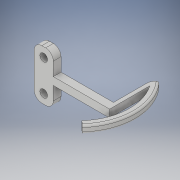
# Autodesk Inventor part: 14HM08 Chassis Sleds
Saved by Autodesk Inventor 2019 (Build 230136000, 136)
## iProperties
Created: 2019-02-17
Part Number: 14HM08 Chassis Sleds
Material: Generic
Document SubType Name: Modeling
Designer: Billy
Density: 1 g/cm^3
Appearance: Default
Author: Billy
Autodesk Inventor part; units mm, degrees
ref_plane "YZ Plane" through (0, 0, 0) normal (1, 0, 0) x (0, 1, 0)
ref_plane "XZ Plane" through (0, 0, 0) normal (0, 1, 0) x (-1, 0, 0)
ref_plane "XY Plane" through (0, 0, 0) normal (0, 0, 1) x (1, 0, 0)
sketch "Sketch1" plane through (0, 0, 0) normal (0, 1, 0) x (-1, 0, 0)
  arc A0 (-22.3607, 20) -> (-22.3607, -20) centre (0, 0) ccw
  arc A1 (-20.1246, 18) -> (-22, -15.6525) centre (0, 0) ccw
  line L0 (-22.3607, -20) -> (0, 0)
  line L1 (-20.1246, 18) -> (-22.3607, 20)
  line L2 (0, 4.0249) -> (-22, -15.6525)
  line L3 (0, 0) -> (8.25, 0)
  line L4 (8.25, 4.0249) -> (0, 4.0249)
  line L5 (8.25, 0) -> (16.25, 0)
  line L6 (16.25, 0) -> (16.25, 4.0249)
  line L7 (16.25, 4.0249) -> (8.25, 4.0249)
  dimension "d4" = 8.25
  dimension "d5" = 8
  constraints: 16 end point, 4 point on circle, 2 centre point, 2 coincident, 2 horizontal, 2 parallel, 1 perpendicular
  measures "d4" distance of L4.start L2.start
  measures "d5" distance of L4.start L6.end
extrude "Extrusion1" add sketch "Sketch1" along normal blind 4
sketch "Sketch2" plane through (-16.25, 0, 4.0249) normal (0, 0, 1) x (1, 0, 0)
  line L0 (16.25, 0) -> (0, 0) projected
  line L1 (16.25, 0) -> (16.25, 4) projected
  line L2 (0, 4) -> (16.25, 4) projected
  line L3 (0, 0) -> (0, 4) projected
  line L4 (0, 4) -> (8, 4)
  line L5 (8, 4) -> (8, 14)
  line L6 (8, 14) -> (0, 14)
  line L7 (0, 14) -> (0, 4)
  line L8 (0, 0) -> (8, 0)
  line L9 (8, 0) -> (8, -10)
  line L10 (8, -10) -> (0, -10)
  line L11 (0, -10) -> (0, 0)
  dimension "d8" = 8
  dimension "d9" = 10
  dimension "d10" = 10
  constraints: 16 end point, 4 parallel, 2 horizontal, 2 perpendicular, 1 point on line
  measures "d8" distance of L6.end L5.end
  measures "d9" distance of L5.end L4.end
  measures "d10" distance of L8.end L9.end
extrude "Extrusion2" add sketch "Sketch2" against normal up to surface (4.0249 mm away) contours L9 L10 L11 L0 | L2 L7 L6 L5
move faces "Move1" translate (0, 0, 1.5) faces at (-13.5833, 2.6667, 0)
sketch "Sketch3" plane through (-16.25, 14, 4.0249) normal (0, 0, 1) x (1, 0, 0)
  line L0 (8, -10) -> (16.25, -10) projected
  line L1 (8, -10) -> (8, 0) projected
  line L2 (8, 0) -> (0, 0) projected
  line L3 (0, 0) -> (0, -24) projected
  line L4 (0, -24) -> (8, -24) projected
  line L5 (8, -24) -> (8, -14) projected
  line L6 (16.25, -14) -> (8, -14) projected
  line L7 (4, -12) -> (4, -20.13)
  line L8 (4, -12) -> (4, -3.87)
  line L9 (4, -12) -> (12.13, -12) construction
  circle A0 centre (4, -3.87) radius 2
  circle A1 centre (4, -20.13) radius 2
  line L10 (16.25, -14) -> (16.25, -10) projected
  dimension "d17" = 8.13
  dimension "d18" = 8.13
  dimension "d19" = 90
  dimension "d20" = 4
  dimension "d21" = 4
  constraints: 6 end point, 2 centre point, 2 coincident, 2 vertical, 1 horizontal, 1 perpendicular
  measures "d17" distance of L7.start L7.end
  measures "d18" distance of L7.start L8.end
  measures "d19" angle of L9 L8
  measures "d20" diameter of A0
  measures "d21" diameter of A1
extrude "Extrusion3" cut sketch "Sketch3" against normal blind 4.1 contours A0 | A1
fillet "Fillet2" radius 3 4 edges at (-16.25, 14, 2.7625) (-8.25, 14, 2.7625) (-16.25, -10, 2.7625) (-8.25, -10, 2.7625)
fillet "Fillet3" radius 1 2 edges at (30, 4, 0) (30, 0, 0)
sketch "Sketch4" plane through (0, 4, 0) normal (0, 1, 0) x (1, 0, 0)
  arc A0 (21.6153, -19.3333) -> (21.6153, 19.3333) centre (0, 0) ccw
  line L0 (20.1246, 18) -> (-1.6771, -1.5)
  line L1 (-8.25, -1.5) -> (-8.25, -4.0249)
  line L2 (-1.6771, -4.0249) -> (0, -4.0249)
  line L3 (0, -4.0249) -> (22, 15.6525)
  arc A1 (20.1246, -18) -> (26.6983, -4.0249) centre (0, 0) ccw
  line L4 (20.1246, -18) -> (21.6153, -19.3333)
  arc A2 (22, 15.6525) -> (20.1246, 18) centre (0, 0) ccw
  line L5 (-1.6771, -1.5) -> (-1.6771, -4.0249)
  constraints: 12 end point, 6 point on circle, 4 centre point, 1 coincident, 1 point on line
extrude "Extrusion4" cut sketch "Sketch4" against normal blind 4.1
sketch "Sketch5" plane through (0, 4, 0) normal (0, 1, 0) x (1, 0, 0)
  arc A0 (20.1246, -18) -> (20.1246, 18) centre (0, 0) ccw projected
  line L0 (20.1246, -18) -> (21.6153, -19.3333) projected
  arc A1 (21.6153, -19.3333) -> (21.6153, 19.3333) centre (0, 0) ccw projected
  line L1 (21.6153, 19.3333) -> (20.1246, 18) projected
  line L2 (-1.6771, -4.0249) -> (-1.6771, -1.5) projected
  line L3 (-1.6771, -1.5) -> (-8.25, -1.5) projected
  line L4 (-8.25, -1.5) -> (-8.25, -4.0249) projected
  line L5 (-8.25, -4.0249) -> (-1.6771, -4.0249) projected
  line L6 (-1.6771, -4.0249) -> (20.1246, -4.0249)
  line L7 (20.1246, -1.5) -> (-1.6771, -1.5)
  line L8 (-1.6771, -1.5) -> (-1.6771, -4.0249)
  arc A2 (20.1246, -18) -> (20.1246, 18) centre (0, 0) ccw projected
  line L9 (20.1246, -4.0249) -> (22.1246, -4.0249)
  line L10 (22.1246, -4.0249) -> (22.1246, 15.4758)
  line L11 (20.1246, 18) -> (20.1246, -1.5)
  constraints: 12 end point, 2 horizontal, 2 parallel, 1 perpendicular, 1 point on circle, 1 point on line
extrude "Extrusion5" add sketch "Sketch5" against normal up to surface (4 mm away) contours L10 L9 L6 L2 L7 L11 A0
fillet "Fillet5" radius 5 1 edges at (20.1246, 2, -18)
move faces "Move4" translate (0, 0, 1.5) faces at (1.8749, 2.6667, 4.0249)
sketch "Sketch6" plane through (-13.25, 14, 5.5249) normal (0, 0, 1) x (1, 0, 0)
  circle A0 centre (1, -20.13) radius 2
  circle A1 centre (1, -3.87) radius 2
  line L0 (5, -10) -> (35.3746, -10) projected
  line L1 (5, -10) -> (5, -3)
  arc A2 (5, -3) -> (2, 0) centre (2, -3) ccw
  line L2 (2, 0) -> (0, 0)
  arc A3 (0, 0) -> (-3, -3) centre (0, -3) ccw
  line L3 (-3, -3) -> (-3, -21)
  arc A4 (-3, -21) -> (0, -24) centre (0, -21) ccw
  line L4 (0, -24) -> (2, -24)
  arc A5 (2, -24) -> (5, -21) centre (2, -21) ccw
  line L5 (5, -21) -> (5, -14)
  line L6 (35.3746, -14) -> (5, -14) projected
  line L7 (35.3746, -10) -> (35.3746, -14) projected
  line L8 (6, -9) -> (6, -21)
  arc A6 (2, -25) -> (6, -21) centre (2, -21) ccw
  line L9 (2, -25) -> (0, -25)
  arc A7 (-4, -21) -> (0, -25) centre (0, -21) ccw
  line L10 (-4, -21) -> (-4, -3)
  arc A8 (0, 1) -> (-4, -3) centre (0, -3) ccw
  line L11 (0, 1) -> (2, 1)
  arc A9 (6, -3) -> (2, 1) centre (2, -3) ccw
  line L12 (6, -3) -> (6, -9)
  line L13 (36.3746, -9) -> (36.3746, -15)
  point P0 (13.25, -14)
  dimension "d42" = 1
  constraints: 22 end point, 16 point on circle, 15 centre point
  measures "d42" distance between parallel lines of L5 L8
extrude "Extrusion6" add sketch "Sketch6" against normal up to surface (4.0249 mm away) contours L1 A2 L2 A3 L3 A4 L4 A5 L5 L6 L8 A6 L9 A7 L10 A8 L11 A9 L12 L0 | L0 L8 L6 L5 A5 L4 A4 L3 A3 L2 A2 L1
body "Solid1"
